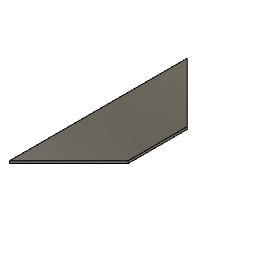
halefinne v0 v1 (Autodesk Fusion 360 design; units mm, degrees)
Autodesk Fusion 360 part; units mm, degrees
sketch "Sketch1" plane through (0, 0, 0) normal (0, 0, 1) x (1, 0, 0)
  line L0 (0, 50) -> (0, -100)
  line L1 (0, 0) -> (50, 0)
  line L2 (50, 0) -> (50, -50)
  line L3 (50, -50) -> (0, -50)
  spline S0 degree 5 poles (0, -100) (2, -98) (6, -94) (12, -88) (20, -80) (30, -70) (38, -62) (44, -56) (48, -52) (50, -50) knots 0 0 0 0 0 0 0.2 0.4 0.6 0.8 1 1 1 1 1 1
  spline S1 degree 5 poles (50, 0) (48, 2) (44, 6) (38, 12) (30, 20) (20, 30) (12, 38) (6, 44) (2, 48) (0, 50) knots 0 0 0 0 0 0 0.2 0.4 0.6 0.8 1 1 1 1 1 1
  constraint vertical L0
  constraint coincident L1.start origin
  constraint perpendicular L0 L1
  constraint perpendicular L1 L2
  constraint coincident L0 L3.end
  constraint perpendicular L0 L3
extrude "Extrude1" add sketch "Sketch1" along normal blind 2
sketch "Sketch2" plane through (0, 0, 0) normal (0, 1, 0) x (1, 0, 0)
